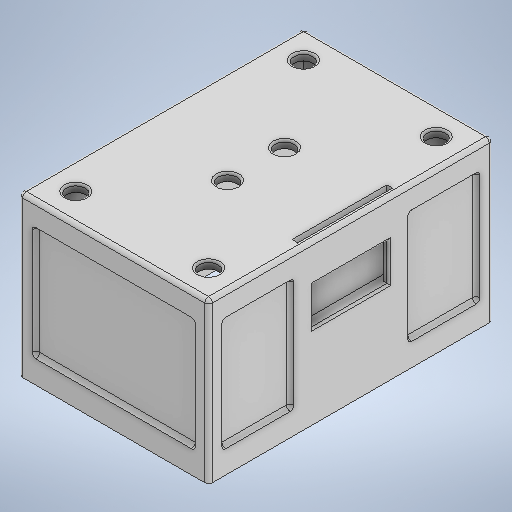
# Autodesk Inventor part: cover-1
Saved by Autodesk Inventor 2025 (Build 290162000, 162)
## iProperties
Created: 2026-01-28
Part Number: cover-1
Material: 一般
Document SubType Name: Modeling
Designer: mahhy
Density: 1 g/cm^3
Appearance: 既定
Author: mahhy
## iProperties of the stored document cover-1_3D プリント.ipt
Created: 2026-01-28
Part Number: cover-1_3D プリント
Material: 一般
Document SubType Name: Modeling
Designer: mahhy
Density: 1 g/cm^3
Appearance: 既定
Author: mahhy
Autodesk Inventor part; units mm, degrees
ref_plane "YZ Plane" through (0, 0, 0) normal (1, 0, 0) x (0, 1, 0)
ref_plane "XZ Plane" through (0, 0, 0) normal (0, 1, 0) x (-1, 0, 0)
ref_plane "XY Plane" through (0, 0, 0) normal (0, 0, 1) x (1, 0, 0)
sketch "スケッチ1" plane through (0, 0, 0) normal (0, 1, 0) x (-1, 0, 0)
  line L0 (0, 0) -> (100, 0)
  line L1 (100, 0) -> (100, -150)
  line L2 (100, -150) -> (0, -150)
  line L3 (0, -150) -> (0, 0)
  line L4 (96, -150) -> (96, -5)
  line L5 (95, -4) -> (5, -4)
  line L6 (4, -5) -> (4, -150)
  arc A0 (96, -5) -> (95, -4) centre (95, -5) ccw
  arc A1 (5, -4) -> (4, -5) centre (5, -5) ccw
  dimension "d0" = 150
  dimension "d1" = 100
  dimension "d2" = 4
  dimension "d3" = 4
  dimension "d4" = 4
  dimension "d5" = 1
  constraints: 14 end point, 4 point on circle, 4 tangent, 3 perpendicular, 2 centre point, 2 parallel, 2 point on line, 1 equal radius, 1 horizontal, 1 vertical
  measures "d0" distance of L0.end L1.end
  measures "d1" distance of L0.start L0.end
  measures "d2" distance between parallel lines of L3 L6
  measures "d3" distance between parallel lines of L1 L4
  measures "d4" distance between parallel lines of L0 L5
  measures "d5" radius of A0
extrude "側面" add sketch "スケッチ1" along normal blind 80 contours L0 L1 L2 L4 A0 L5 A1 L6 L3
sketch "スケッチ2" plane through (0, 80, 0) normal (0, 1, 0) x (1, 0, 0)
  line L0 (-100, 0) -> (0, 0) projected
  line L1 (0, 150) -> (-4, 150) projected
  line L2 (-100, 0) -> (0, 0)
  line L3 (0, 0) -> (0, 150)
  line L4 (0, 150) -> (-100, 150)
  line L5 (-100, 150) -> (-100, 0)
  constraints: 8 end point, 2 parallel, 1 horizontal, 1 perpendicular
extrude "上面" add sketch "スケッチ2" along normal blind 4
sketch "スケッチ3" plane through (0, 0, 0) normal (0, -1, 0) x (1, 0, 0)
  line L0 (-4, -150) -> (-4, -5) projected
  line L1 (-4, -105) -> (-9, -105)
  line L2 (-9, -105) -> (-9, -110)
  line L3 (-9, -110) -> (-4, -110)
  line L4 (-4, -110) -> (-4, -105)
  line L5 (-96, -5) -> (-96, -150) projected
  line L6 (-96, -74.5) -> (-91, -74.5)
  line L7 (-91, -74.5) -> (-91, -79.5)
  line L8 (-91, -79.5) -> (-96, -79.5)
  line L9 (-96, -79.5) -> (-96, -74.5)
  line L10 (-4, -44) -> (-9, -44)
  line L11 (-9, -44) -> (-9, -49)
  line L12 (-9, -49) -> (-4, -49)
  line L13 (-4, -49) -> (-4, -44)
  line L14 (-5, -4) -> (-95, -4) projected
  line L15 (-4, -150) -> (-96, -150) projected
  point P0 (0, 0)
  point P1 (-9, -46.5)
  point P2 (-9, -107.5)
  point P3 (-4, -110)
  point P4 (-96, -79.5)
  dimension "d11" = 5
  dimension "d12" = 40
  dimension "d13" = 5
  dimension "d14" = 56
  dimension "d15" = 5
  dimension "d16" = 5
  dimension "d17" = 5
  dimension "d97" = 70.5
  constraints: 24 end point, 6 parallel, 3 horizontal, 3 perpendicular, 3 point on line, 2 midpoint, 1 vertical alignment
  measures "d11" distance of L6.end L7.end
  measures "d12" distance between parallel lines of L14 L10
  measures "d13" distance of L10.end L11.end
  measures "d14" distance between parallel lines of L12 L1
  measures "d15" distance of L1.end L2.end
  measures "d16" distance between parallel lines of L0 L11
  measures "d17" distance between parallel lines of L5 L7
  measures "d97" distance between parallel lines of L15 L8
extrude "接合部" add sketch "スケッチ3" against normal blind 80
sketch "スケッチ4" plane through (0, 80, 0) normal (0, -1, 0) x (1, 0, 0)
  line L0 (-4, -150) -> (-4, -110) projected
  line L1 (-4, -150) -> (-96, -150)
  line L2 (-96, -150) -> (-96, -146)
  line L3 (-96, -146) -> (-4, -146)
  line L4 (-4, -146) -> (-4, -150)
  line L5 (-96, -79.5) -> (-96, -150) projected
  point P0 (0, 0)
  point P1 (-96, -148)
  point P2 (-4, -146)
  dimension "d21" = 4
  constraints: 8 end point, 2 parallel, 1 horizontal, 1 midpoint, 1 perpendicular, 1 point on line
  measures "d21" distance of L1.end L2.end
extrude "側面2" add sketch "スケッチ4" along normal blind 75
sketch "スケッチ5" plane through (0, 84, 0) normal (0, 1, 0) x (1, 0, 0)
  circle A0 centre (-15, 15) radius 5
  circle A1 centre (-15, 135) radius 5
  circle A2 centre (-85, 135) radius 5
  circle A3 centre (-85, 15) radius 5
  circle A4 centre (-50, 60) radius 5
  circle A5 centre (-50, 90) radius 5
  line L0 (0, 0) -> (0, 150) projected
  line L1 (0, 75) -> (-100, 75)
  line L2 (-100, 150) -> (-100, 0) projected
  line L3 (-100, 0) -> (0, 0) projected
  line L4 (0, 150) -> (-100, 150) projected
  point P0 (-50, 75)
  dimension "d24" = 10
  dimension "d25" = 10
  dimension "d26" = 10
  dimension "d27" = 10
  dimension "d28" = 10
  dimension "d29" = 10
  dimension "d30" = 15
  dimension "d31" = 15
  dimension "d32" = 15
  dimension "d33" = 15
  dimension "d34" = 15
  dimension "d35" = 15
  constraints: 6 centre point, 4 vertical alignment, 3 midpoint, 2 end point, 2 horizontal alignment
  measures "d24" diameter of A0
  measures "d25" diameter of A1
  measures "d26" diameter of A2
  measures "d27" diameter of A3
  measures "d28" diameter of A4
  measures "d29" diameter of A5
  measures "d30" distance from line of L1 A4.centre
  measures "d31" distance from line of L3 A0.centre
  measures "d32" distance from line of L1 A5.centre
  measures "d33" distance from line of L4 A1.centre
  measures "d34" distance from line of L0 A0.centre
  measures "d35" distance from line of L2 A3.centre
extrude "はめ込み穴" cut sketch "スケッチ5" against normal through all contours A0 | A1 | A2 | A3 | A4 | A5
sketch "スケッチ7" plane through (0, 80, 0) normal (0, -1, 0) x (1, 0, 0)
  line L0 (-4, -105) -> (-4, -49) projected
  line L1 (-4, -45) -> (-9, -45)
  line L2 (-9, -45) -> (-9, -105)
  line L3 (-9, -105) -> (-4, -105)
  line L4 (-4, -105) -> (-4, -45)
  line L5 (0, 0) -> (0, -150) projected
  point P0 (-9, -75)
  point P1 (0, -75)
  dimension "d40" = 5
  dimension "d41" = 60
  constraints: 8 end point, 2 midpoint, 2 parallel, 1 horizontal, 1 horizontal alignment, 1 perpendicular, 1 point on line
  measures "d40" distance of L3.end L2.end
  measures "d41" distance of L2.end L1.end
extrude "押し出し6" add sketch "スケッチ7" along normal blind 50
sketch "スケッチ8" plane through (0, 84, 0) normal (0, 1, 0) x (1, 0, 0)
  line L0 (-29.5069, 279.0515) -> (-42.6104, 279.0515)
  line L1 (-42.6104, 279.0515) -> (-42.6104, 309.0515)
  line L2 (-42.6104, 309.0515) -> (-29.5069, 309.0515)
  line L3 (-29.5069, 309.0515) -> (-29.5069, 279.0515)
  line L4 (-3, 50) -> (-6, 50)
  line L5 (-6, 50) -> (-6, 100)
  line L6 (-6, 100) -> (-3, 100)
  line L7 (-3, 100) -> (-3, 50)
  line L8 (0, 0) -> (0, 150) projected
  line L9 (0, 62.5) -> (-3, 62.5)
  line L10 (-3, 62.5) -> (-3, 87.5)
  line L11 (-3, 87.5) -> (0, 87.5)
  line L12 (0, 87.5) -> (0, 62.5)
  point P0 (0, 75)
  point P1 (0, 75)
  point P2 (-6, 75)
  point P3 (0, 75)
  dimension "d44" = 30
  dimension "d45" = 25
  dimension "d46" = 50
  dimension "d47" = 3
  dimension "d48" = 3
  constraints: 24 end point, 6 parallel, 4 midpoint, 3 horizontal, 3 perpendicular, 2 point on line, 1 coincident, 1 horizontal alignment
  measures "d44" distance of L0.end L1.end
  measures "d45" distance from line of L11.end L9
  measures "d46" distance of L6.end L4.start
  measures "d47" distance of L9.start L9.end
  measures "d48" distance of L4.start L4.end
extrude "押し出し7" cut sketch "スケッチ8" against normal blind 40 contours L4 L5 L6 L7
sketch "スケッチ9" plane through (0, 0, 0) normal (1, 0, 0) x (0, 0, -1)
  line L0 (55, 44) -> (95, 44)
  line L1 (95, 44) -> (95, 64)
  line L2 (95, 64) -> (55, 64)
  line L3 (55, 64) -> (55, 44)
  line L4 (0, 84) -> (150, 84) projected
  point P0 (0, 0)
  point P1 (75, 64)
  point P2 (75, 84)
  dimension "d51" = 40
  dimension "d52" = 20
  dimension "d53" = 20
  constraints: 8 end point, 2 midpoint, 2 parallel, 1 horizontal, 1 perpendicular, 1 vertical alignment
  measures "d51" distance of L2.end L1.end
  measures "d52" distance of L2.end L0.start
  measures "d53" distance between parallel lines of L4 L2
extrude "押し出し8" cut sketch "スケッチ9" against normal blind 5
fillet "フィレット1" radius 2 10 edges at (0, 42, 0) (-50, 84, 0) (-100, 84, -75) (-50, 84, -150) (0, 42, -150) (0, 84, -75) (-100, 42, -150) (-100, 42, 0) (-9, 30, -77) (-4, 30, -77)
fillet "フィレット2" radius 1 6 edges at (-90, 84, -15) (-20, 84, -15) (-55, 84, -60) (-55, 84, -90) (-20, 84, -135) (-90, 84, -135)
fillet "フィレット3" radius 1 4 edges at (0, 44, -75) (0, 54, -55) (0, 64, -75) (0, 54, -95)
sketch "スケッチ10" plane through (-100, 0, -148) normal (-1, 0, 0) x (0, 0, 1)
  line L0 (7, 72) -> (139, 72)
  line L1 (141, 70) -> (141, 14)
  line L2 (139, 12) -> (7, 12)
  line L3 (5, 14) -> (5, 70)
  line L4 (146, 82) -> (146, 0) projected
  line L5 (0, 82) -> (146, 82) projected
  line L6 (0, 0) -> (146, 0) projected
  line L7 (0, 0) -> (0, 82) projected
  line L8 (146, 84) -> (0, 84) projected
  line L9 (148, 0) -> (148, 82) projected
  line L10 (-2, 82) -> (-2, 0) projected
  arc A0 (7, 72) -> (5, 70) centre (7, 70) ccw
  arc A1 (5, 14) -> (7, 12) centre (7, 14) ccw
  arc A2 (139, 12) -> (141, 14) centre (139, 14) ccw
  arc A3 (141, 70) -> (139, 72) centre (139, 70) ccw
  point P0 (5, 72)
  point P1 (141, 12)
  point P2 (141, 72)
  point P3 (5, 12)
  dimension "d61" = 12
  dimension "d63" = 12
  dimension "d64" = 7
  dimension "d65" = 7
  dimension "d94" = 2
  constraints: 8 end point, 8 point on circle, 8 point on line, 8 tangent, 4 centre point, 3 equal radius, 2 parallel, 1 horizontal, 1 perpendicular
  measures "d61" distance between parallel lines of L6 L2
  measures "d63" distance between parallel lines of L8 L0
  measures "d64" distance between parallel lines of L9 L1
  measures "d65" distance between parallel lines of L10 L3
  measures "d94" radius of A0
extrude "押し出し9" cut sketch "スケッチ10" against normal blind 2 contours L0 A3 L1 A2 L2 A1 L3 A0
sketch "スケッチ11" plane through (-98, 0, 0) normal (0, 0, 1) x (1, 0, 0)
  line L0 (7, 72) -> (89, 72)
  line L1 (91, 70) -> (91, 14)
  line L2 (89, 12) -> (7, 12)
  line L3 (5, 14) -> (5, 70)
  line L4 (98, 0) -> (98, 82) projected
  line L5 (96, 84) -> (0, 84) projected
  line L6 (0, 0) -> (96, 0) projected
  line L7 (-2, 82) -> (-2, 0) projected
  arc A0 (7, 72) -> (5, 70) centre (7, 70) ccw
  arc A1 (91, 70) -> (89, 72) centre (89, 70) ccw
  arc A2 (89, 12) -> (91, 14) centre (89, 14) ccw
  arc A3 (5, 14) -> (7, 12) centre (7, 14) ccw
  point P0 (5, 72)
  point P1 (91, 12)
  point P2 (91, 72)
  point P3 (5, 12)
  dimension "d69" = 7
  dimension "d70" = 12
  dimension "d71" = 12
  dimension "d72" = 7
  dimension "d95" = 2
  constraints: 8 end point, 8 point on circle, 8 point on line, 8 tangent, 4 centre point, 3 equal radius, 2 parallel, 1 horizontal, 1 perpendicular
  measures "d69" distance between parallel lines of L4 L1
  measures "d70" distance between parallel lines of L5 L0
  measures "d71" distance between parallel lines of L6 L2
  measures "d72" distance between parallel lines of L7 L3
  measures "d95" radius of A0
extrude "押し出し10" cut sketch "スケッチ11" against normal blind 2
sketch "スケッチ12" plane through (0, 0, -2) normal (1, 0, 0) x (0, 0, -1)
  line L0 (7, 72) -> (41, 72)
  line L1 (43, 70) -> (43, 14)
  line L2 (41, 12) -> (7, 12)
  line L3 (5, 14) -> (5, 70)
  line L4 (105, 72) -> (139, 72)
  line L5 (141, 70) -> (141, 14)
  line L6 (139, 12) -> (105, 12)
  line L7 (103, 14) -> (103, 70)
  line L8 (-2, 82) -> (-2, 0) projected
  line L9 (53, 44) -> (53, 64) projected
  line L10 (146, 84) -> (0, 84) projected
  line L11 (0, 0) -> (146, 0) projected
  line L12 (93, 64) -> (93, 44) projected
  line L13 (148, 0) -> (148, 82) projected
  arc A0 (7, 72) -> (5, 70) centre (7, 70) ccw
  arc A1 (43, 70) -> (41, 72) centre (41, 70) ccw
  arc A2 (41, 12) -> (43, 14) centre (41, 14) ccw
  arc A3 (5, 14) -> (7, 12) centre (7, 14) ccw
  arc A4 (105, 72) -> (103, 70) centre (105, 70) ccw
  arc A5 (141, 70) -> (139, 72) centre (139, 70) ccw
  arc A6 (139, 12) -> (141, 14) centre (139, 14) ccw
  arc A7 (103, 14) -> (105, 12) centre (105, 14) ccw
  point P0 (103, 72)
  point P1 (141, 12)
  dimension "d76" = 7
  dimension "d77" = 10
  dimension "d78" = 12
  dimension "d79" = 12
  dimension "d80" = 10
  dimension "d81" = 7
  dimension "d82" = 2
  constraints: 16 end point, 16 point on circle, 16 tangent, 8 centre point, 7 equal radius, 6 point on line, 4 parallel, 2 horizontal, 2 perpendicular
  measures "d76" distance between parallel lines of L8 L3
  measures "d77" distance between parallel lines of L9 L1
  measures "d78" distance between parallel lines of L10 L0
  measures "d79" distance between parallel lines of L11 L2
  measures "d80" distance between parallel lines of L12 L7
  measures "d81" distance between parallel lines of L13 L5
  measures "d82" radius of A0
extrude "押し出し11" cut sketch "スケッチ12" against normal blind 2
sketch "スケッチ13" plane through (-4, 5, -150) normal (0, 0, -1) x (-1, 0, 0)
  line L0 (91, -5) -> (91, 75) projected
  line L1 (92, 0) -> (0, 0) projected
  line L2 (1, -5) -> (91, -5) projected
  line L3 (5, 67) -> (87, 67)
  line L4 (89, 65) -> (89, 9)
  line L5 (87, 7) -> (5, 7)
  line L6 (3, 9) -> (3, 65)
  line L7 (94, 79) -> (-2, 79) projected
  line L8 (96, -5) -> (96, 77) projected
  line L9 (-4, 77) -> (-4, -5) projected
  arc A0 (5, 67) -> (3, 65) centre (5, 65) ccw
  arc A1 (3, 9) -> (5, 7) centre (5, 9) ccw
  arc A2 (89, 65) -> (87, 67) centre (87, 65) ccw
  arc A3 (87, 7) -> (89, 9) centre (87, 9) ccw
  point P0 (3, 67)
  point P1 (89, 7)
  point P2 (89, 67)
  point P3 (3, 7)
  dimension "d89" = 12
  dimension "d90" = 12
  dimension "d91" = 7
  dimension "d92" = 7
  dimension "d93" = 2
  constraints: 8 end point, 8 point on circle, 8 point on line, 8 tangent, 4 centre point, 3 equal radius, 2 parallel, 1 horizontal, 1 perpendicular
  measures "d89" distance between parallel lines of L7 L3
  measures "d90" distance between parallel lines of L2 L5
  measures "d91" distance between parallel lines of L8 L4
  measures "d92" distance between parallel lines of L9 L6
  measures "d93" radius of A0
extrude "押し出し12" cut sketch "スケッチ13" against normal blind 2
fillet "フィレット6" radius 2 40 edges at (-92.4142, 12.5858, -2) (-93, 42, -2) (-92.4142, 71.4142, -2) (-50, 72, -2) (-7.5858, 71.4142, -2) (-7, 42, -2) (-7.5858, 12.5858, -2) (-50, 12, -2) (-98, 12.5858, -142.4142) (-98, 42, -143) (-98, 71.4142, -142.4142) (-98, 72, -75) (-98, 71.4142, -7.5858) (-98, 42, -7) (-98, 12.5858, -7.5858) (-98, 12, -75) (-7.5858, 12.5858, -148) (-7, 42, -148) (-7.5858, 71.4142, -148) (-50, 72, -148) (-92.4142, 71.4142, -148) (-93, 42, -148) (-92.4142, 12.5858, -148) (-50, 12, -148) (-2, 12.5858, -105.5858) (-2, 42, -105) (-2, 71.4142, -105.5858) (-2, 72, -124) (-2, 71.4142, -142.4142) (-2, 42, -143) (-2, 12.5858, -142.4142) (-2, 12, -124) (-2, 12.5858, -7.5858) (-2, 42, -7) (-2, 71.4142, -7.5858) (-2, 72, -26) (-2, 71.4142, -44.4142) (-2, 42, -45) (-2, 12.5858, -44.4142) (-2, 12, -26)
equation "\"d3\" = d2"
equation "\"d4\" = d2"
equation "\"d11\" = d13"
equation "\"d15\" = d13"
equation "\"d17\" = d16"
equation "\"d25\" = d24"
equation "\"d26\" = d24"
equation "\"d27\" = d24"
equation "\"d28\" = d24"
equation "\"d29\" = d24"
equation "\"d31\" = d30"
equation "\"d32\" = d30"
equation "\"d33\" = d30"
equation "\"d34\" = d30"
equation "\"d35\" = d30"
equation "\"d61\" = d63"
equation "\"d65\" = d64"
equation "\"d71\" = d70"
equation "\"d72\" = d69"
equation "\"d80\" = d77"
equation "\"d81\" = d76"
equation "\"d90\" = d89"
